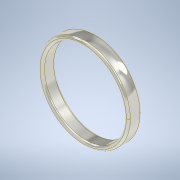
# Autodesk Inventor part: Кольцо
Saved by Autodesk Inventor 2020 (Build 240168000, 168)
## iProperties
Created: 2021-11-26
Part Number: Кольцо
Material: Серебро
Document SubType Name: Modeling
Designer: Анастасия
Density: 10.49 g/cm^3
Appearance: Серебро
Author: Анастасия
Autodesk Inventor part; units mm, degrees
ref_plane "YZ Plane" through (0, 0, 0) normal (1, 0, 0) x (0, 1, 0)
ref_plane "XZ Plane" through (0, 0, 0) normal (0, 1, 0) x (-1, 0, 0)
ref_plane "XY Plane" through (0, 0, 0) normal (0, 0, 1) x (1, 0, 0)
sketch "Эскиз1" plane through (0, 0, 0) normal (0, 0, 1) x (1, 0, 0)
  circle A0 centre (0, 0) radius 20
  circle A1 centre (0, 0) radius 18
  line L0 (0, -20) -> (0, 20)
  point P0 (0, 18)
  point P1 (0, -18)
  dimension "d0" = 20
  dimension "d1" = 18
  constraints: 3 coincident, 2 centre point, 2 end point, 2 point on circle, 1 midpoint, 1 vertical
  measures "d0" radius of A0
  measures "d1" radius of A1
revolve "Вращение1" add sketch "Эскиз1" angle 360 about axis through (0, -20, 0) along (0, 1, 0) picked at (-3.0313, -18.9653) contours L0 A1 A0
sketch "Эскиз2" plane through (0, 0, 0) normal (0, 0, 1) x (1, 0, 0)
  circle A0 centre (0, 0) radius 18
  dimension "d3" = 18
  constraints: 1 centre point, 1 coincident
  measures "d3" radius of A0
extrude "Выдавливание1" cut sketch "Эскиз2" along normal mid plane 50
sketch "Эскиз3" plane through (0, 0, 0) normal (1, 0, 0) x (0, 1, 0)
  arc A0 (-18, 8.7178) -> (18, 8.7178) centre (0, 0) ccw projected
  line L0 (19.7737, 3) -> (-19.7737, 3)
  line L1 (19.7737, -3) -> (-19.7737, -3)
  line L2 (-18, 8.7178) -> (18, 8.7178) projected
  line L3 (18, 8.7178) -> (-18, 8.7178)
  line L4 (18, -8.7178) -> (18, 8.7178) projected
  line L5 (18, -8.7178) -> (-18, -8.7178) projected
  line L6 (18, -8.7178) -> (-18, -8.7178)
  dimension "d6" = 6
  dimension "d7" = 3
  constraints: 8 end point, 3 horizontal, 1 point on line, 6 other
  measures "d6" distance between parallel lines of L1 L0
  measures "d7" distance from line of point (0, 0) L0
extrude "Выдавливание2" cut sketch "Эскиз3" along normal mid plane 50 contours L2 L4 L0 A0 | A0 L0 L4 | L1 L4 L5 A0 | L1 A0 L4
fillet "Сопряжение1" radius 1 6 edges at (-18, 0, 3) (-19.7737, 0, 3) (19.7737, 0, 3) (-18, 0, -3) (-19.7737, 0, -3) (19.7737, 0, -3)
